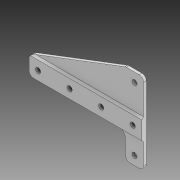
# Autodesk Inventor part: Cart Carrier
Saved by Autodesk Inventor 2020 (Build 240168000, 168)
## iProperties
Created: 2020-10-19
Part Number: Cart Carrier
Material: Generic
Document SubType Name: Modeling
Designer: DDeGo
Density: 1 g/cm^3
Appearance: Default
Author: DDeGo
Autodesk Inventor part; units mm, degrees
ref_plane "YZ Plane" through (0, 0, 0) normal (1, 0, 0) x (0, 1, 0)
ref_plane "XZ Plane" through (0, 0, 0) normal (0, 1, 0) x (-1, 0, 0)
sketch "Sketch1" plane through (0, 0, 0) normal (0, 0, 1) x (1, 0, 0)
  line L0 (-62.5, -10) -> (42.5, -10)
  line L1 (62.5, -10) -> (62.5, 10)
  line L2 (62.5, 10) -> (-62.5, 10) construction
  line L3 (-62.5, 10) -> (-62.5, -10)
  line L4 (-62.5, -10) -> (62.5, 10) construction
  line L5 (62.5, -10) -> (-62.5, 10) construction
  line L6 (62.5, 10) -> (62.5, 50)
  line L7 (62.5, 50) -> (42.5, 50)
  line L8 (62.5, -40) -> (62.5, -10)
  line L9 (-52.5, 10) -> (-52.5, -10) construction
  line L10 (42.5, -40) -> (62.5, -40)
  line L11 (42.5, -40) -> (42.5, -10)
  line L12 (52.5, 50) -> (52.5, -40) construction
  line L13 (-52.5, 0) -> (0, 0) construction
  line L14 (0, 0) -> (52.5, 5) construction
  circle A0 centre (-52.5, 0) radius 2.75
  circle A1 centre (52.5, 40) radius 2.75
  circle A2 centre (52.5, -30) radius 2.75
  line L15 (42.5, -10) -> (42.5, 50) construction
  line L16 (42.5, -10) -> (62.5, -10) construction
  line L17 (-62.5, 10) -> (42.5, 50)
  circle A3 centre (-77.5, 0) radius 10 construction
  line L18 (-77.5, 0) -> (-52.5, 0) construction
  dimension "d8" = 20
  dimension "d9" = 105
  dimension "d13" = 10
  dimension "d14" = 10
  dimension "d15" = 5.5
  dimension "d16" = 10
  dimension "d17" = 10
  dimension "d18" = 10
  dimension "d22" = 40
  dimension "d23" = 30
  dimension "d29" = 20
  dimension "d30" = 130
  constraints: 38 end point, 7 perpendicular, 6 midpoint, 5 horizontal, 4 centre point, 4 point on line, 4 vertical, 3 parallel, 2 equal radius, 1 coincident
  measures "d8" distance of L1.start L1.end
  measures "d9" distance between parallel lines of L12 L9
  measures "d13" distance from line of L10 A2.centre
  measures "d14" distance from line of L7 A1.centre
  measures "d15" diameter of A2
  measures "d16" distance between parallel lines of L8 L12
  measures "d17" distance between parallel lines of L11 L12
  measures "d18" distance between parallel lines of L3 L9
  measures "d22" distance of L1.end L6.end
  measures "d23" distance of L8.start L1.start
  measures "d29" diameter of A3
  measures "d30" distance from line of L12 L18.start
extrude "Extrusion1" add sketch "Sketch1" along normal blind 3
sketch "Sketch4" plane through (0, 0, 3) normal (0, 0, 1) x (1, 0, 0)
  line L0 (-62.5, -10) -> (42.5, -10) projected
  line L1 (-62.5, -10) -> (62.5, -10)
  line L2 (62.5, -10) -> (62.5, 10)
  line L3 (62.5, 10) -> (-62.5, 10)
  line L4 (-62.5, 10) -> (-62.5, -10)
  line L5 (62.5, -40) -> (62.5, 50) projected
  circle A0 centre (-52.5, 0) radius 2.75 projected
  point P0 (0, 0)
  point P1 (-62.5, 10)
  point P2 (42.5, -10)
  constraints: 8 end point, 2 parallel, 1 coincident, 1 horizontal, 1 perpendicular, 1 point on line
extrude "Extrusion4" add sketch "Sketch4" along normal blind 2
fillet "Fillet1" radius 10 1 edges at (42.5, -10, 1.5)
fillet "Fillet1" radius 5 6 edges at (42.5, -40, 1.5) (62.5, -40, 1.5) (-62.5, -10, 2.5) (-62.5, 10, 1.5) (42.5, 50, 1.5) (62.5, 50, 1.5)
sketch "Sketch3" plane through (0, 0, 0) normal (0, 0, -1) x (-1, 0, 0)
  circle A0 centre (-17.5, 0) radius 2.75
  line L0 (57.5, -10) -> (-32.5, -10) projected
  line L1 (-17.5, 0) -> (-52.5, 0) construction
  line L2 (-17.5, 0) -> (17.5, 0) construction
  circle A1 centre (-52.5, 0) radius 2.75
  circle A2 centre (17.5, 0) radius 2.75
  circle A3 centre (52.5, 0) radius 2.75 projected
  line L3 (52.5, 0) -> (17.5, 0) construction
  line L4 (-62.5, -35) -> (-62.5, 45) projected
  point P0 (62.5, -10)
  point P1 (-42.5, -10)
  point P2 (-62.5, -40)
  point P3 (-62.5, 50)
  dimension "d24" = 5.5
  dimension "d31" = 10
  constraints: 6 end point, 3 centre point, 3 coincident, 3 horizontal, 2 collinear, 2 equal radius
  measures "d24" diameter of A0
  measures "d31" distance from line of L4 L1.end
extrude "Extrusion3" cut sketch "Sketch3" against normal through all contours A0 | A1 | A2
chamfer "Chamfer1" distance 2 angle 45 2 edges at (47.5, -10, 3) (0.6885, 10, 3)
ref_plane "Work Plane1" through (46.2681, 37.5241, 3) normal (-0.3559953, 0.9344877, 0) x (0.9344877, 0.3559953, 0)
sketch "Sketch5" plane through (46.2681, 37.5241, 3) normal (-0.3559953, 0.9344877, 0) x (0.9344877, 0.3559953, 0)
  line L0 (0, 3) -> (-107.9951, 3) projected
  line L1 (-97.906, 3) -> (-71.2728, 7.6962)
  line L2 (-67.7998, 8) -> (-31.1511, 8)
  line L3 (6.0821, 0) -> (-105.8228, 0) projected
  line L4 (-27.6782, 7.6962) -> (-1.0449, 3)
  line L5 (-1.0449, 3) -> (-97.906, 3)
  line L6 (9.4551, 3) -> (3.9551, 3) projected
  line L7 (-102.906, 3) -> (-108.406, 3) projected
  arc A0 (-27.6782, 7.6962) -> (-31.1511, 8) centre (-31.1511, -12) ccw
  arc A1 (-67.7998, 8) -> (-71.2728, 7.6962) centre (-67.7998, -12) ccw
  point P0 (-56.5954, 3)
  dimension "d38" = 5
  dimension "d39" = 5
  dimension "d40" = 5
  dimension "d41" = 10
  dimension "d42" = 10
  dimension "d43" = 20
  constraints: 8 end point, 4 point on circle, 4 tangent, 2 centre point, 2 point on line, 1 equal radius, 1 parallel
  measures "d38" distance of L1.start L7.start
  measures "d39" distance of L6.end L4.end
  measures "d40" distance between parallel lines of L2 L0
  measures "d41" angle of L0 L4
  measures "d42" angle of L0 L1
  measures "d43" radius of A0
extrude "Extrusion5" add sketch "Sketch5" along normal mid plane 4
fillet "Fillet2" radius 2 2 edges at (0.7459, 18.0421, 0) (-0.6781, 21.78, 0)
fillet "Fillet2" radius 1 10 edges at (19.4987, 25.186, -4.9239) (33.5594, 30.5425, -2.3481) (-18.0069, 10.8982, -4.9239) (-32.0676, 5.5417, -2.3481) (0.7459, 18.0421, -5) (-19.4309, 14.6361, -4.9239) (-33.4916, 9.2797, -2.3481) (18.0747, 28.924, -4.9239) (32.1354, 34.2804, -2.3481) (-0.6781, 21.78, -5)
equation "\"d14\" = d13"
equation "\"d42\" = d41"
body "Solid1"
